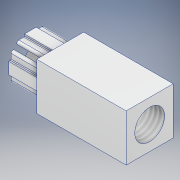
# Autodesk Inventor part: Line 5 Bucket Adapter
Saved by Autodesk Inventor 2020 (Build 240168000, 168)
## iProperties
Created: 2019-10-01
Part Number: Line 5 Bucket Adapter
Material: Aluminum 6061
Document SubType Name: Modeling
Designer: Matt
Density: 2.7 g/cm^3
Appearance: Aluminum - Flat
Mass: 38.6702 g
Surface Area: 66.6995 cm^2
Volume: 14.3223 cm^3
Author: Matt
Autodesk Inventor part; units mm, degrees
ref_plane "YZ Plane" through (0, 0, 0) normal (1, 0, 0) x (0, 1, 0)
ref_plane "XZ Plane" through (0, 0, 0) normal (0, 1, 0) x (-1, 0, 0)
ref_plane "XY Plane" through (0, 0, 0) normal (0, 0, 1) x (1, 0, 0)
sketch "Sketch1" plane through (0, 0, 0) normal (1, 0, 0) x (0, 1, 0)
  arc A0 (3.3, 10) -> (2.5, 9.2) centre (3.3, 9.2) ccw
  line L0 (2.5, 9.2) -> (2.5, 8.5)
  arc A1 (2.5, 8.5) -> (2.8, 8.2) centre (2.8, 8.5) ccw
  line L1 (2.8, 8.2) -> (4.9176, 8.2)
  arc A2 (5.5062, 6.779) -> (4.9176, 8.2) centre (4.9176, 7.3676) ccw
  line L2 (5.5062, 6.779) -> (3.2559, 4.5287)
  arc A3 (1.1346, 3.65) -> (3.2559, 4.5287) centre (1.1346, 6.65) ccw
  line L3 (1.1346, 3.65) -> (-1.1346, 3.65)
  arc A4 (-3.2559, 4.5287) -> (-1.1346, 3.65) centre (-1.1346, 6.65) ccw
  line L4 (-3.2559, 4.5287) -> (-5.5062, 6.779)
  arc A5 (-4.9176, 8.2) -> (-5.5062, 6.779) centre (-4.9176, 7.3676) ccw
  line L5 (-4.9176, 8.2) -> (-2.8, 8.2)
  arc A6 (-2.8, 8.2) -> (-2.5, 8.5) centre (-2.8, 8.5) ccw
  line L6 (-2.5, 8.5) -> (-2.5, 9.2)
  arc A7 (-2.5, 9.2) -> (-3.3, 10) centre (-3.3, 9.2) ccw
  line L7 (-8, 10) -> (-3.3, 10)
  arc A8 (-8, 10) -> (-10, 8) centre (-8, 8) ccw
  line L8 (-10, -3.3) -> (-10, 8)
  arc A9 (-10, 3.3) -> (-9.2, 2.5) centre (-9.2, 3.3) ccw
  line L9 (-9.2, 2.5) -> (-8.5, 2.5)
  arc A10 (-8.5, 2.5) -> (-8.2, 2.8) centre (-8.5, 2.8) ccw
  line L10 (-8.2, 2.8) -> (-8.2, 4.9176)
  arc A11 (-6.779, 5.5062) -> (-8.2, 4.9176) centre (-7.3676, 4.9176) ccw
  line L11 (-6.779, 5.5062) -> (-4.5287, 3.2559)
  arc A12 (-3.65, 1.1346) -> (-4.5287, 3.2559) centre (-6.65, 1.1346) ccw
  line L12 (-3.65, 1.1346) -> (-3.65, -1.1346)
  arc A13 (-4.5287, -3.2559) -> (-3.65, -1.1346) centre (-6.65, -1.1346) ccw
  line L13 (-4.5287, -3.2559) -> (-6.779, -5.5062)
  arc A14 (-8.2, -4.9176) -> (-6.779, -5.5062) centre (-7.3676, -4.9176) ccw
  line L14 (-8.2, -4.9176) -> (-8.2, -2.8)
  arc A15 (-8.2, -2.8) -> (-8.5, -2.5) centre (-8.5, -2.8) ccw
  line L15 (-8.5, -2.5) -> (-9.2, -2.5)
  arc A16 (-9.2, -2.5) -> (-10, -3.3) centre (-9.2, -3.3) ccw
  line L16 (-10, -8) -> (-10, -3.3)
  arc A17 (-10, -8) -> (-8, -10) centre (-8, -8) ccw
  line L17 (3.3, -10) -> (-8, -10)
  arc A18 (-3.3, -10) -> (-2.5, -9.2) centre (-3.3, -9.2) ccw
  line L18 (-2.5, -9.2) -> (-2.5, -8.5)
  arc A19 (-2.5, -8.5) -> (-2.8, -8.2) centre (-2.8, -8.5) ccw
  line L19 (-2.8, -8.2) -> (-4.9176, -8.2)
  arc A20 (-5.5062, -6.779) -> (-4.9176, -8.2) centre (-4.9176, -7.3676) ccw
  line L20 (-5.5062, -6.779) -> (-3.2559, -4.5287)
  arc A21 (-1.1346, -3.65) -> (-3.2559, -4.5287) centre (-1.1346, -6.65) ccw
  line L21 (-1.1346, -3.65) -> (1.1346, -3.65)
  arc A22 (3.2559, -4.5287) -> (1.1346, -3.65) centre (1.1346, -6.65) ccw
  line L22 (3.2559, -4.5287) -> (5.5062, -6.779)
  arc A23 (4.9176, -8.2) -> (5.5062, -6.779) centre (4.9176, -7.3676) ccw
  line L23 (4.9176, -8.2) -> (2.8, -8.2)
  arc A24 (2.8, -8.2) -> (2.5, -8.5) centre (2.8, -8.5) ccw
  line L24 (2.5, -8.5) -> (2.5, -9.2)
  arc A25 (2.5, -9.2) -> (3.3, -10) centre (3.3, -9.2) ccw
  line L25 (8, -10) -> (3.3, -10)
  arc A26 (8, -10) -> (10, -8) centre (8, -8) ccw
  line L26 (10, 3.3) -> (10, -8)
  arc A27 (10, -3.3) -> (9.2, -2.5) centre (9.2, -3.3) ccw
  line L27 (9.2, -2.5) -> (8.5, -2.5)
  arc A28 (8.5, -2.5) -> (8.2, -2.8) centre (8.5, -2.8) ccw
  line L28 (8.2, -2.8) -> (8.2, -4.9176)
  arc A29 (6.779, -5.5062) -> (8.2, -4.9176) centre (7.3676, -4.9176) ccw
  line L29 (6.779, -5.5062) -> (4.5287, -3.2559)
  arc A30 (3.65, -1.1346) -> (4.5287, -3.2559) centre (6.65, -1.1346) ccw
  line L30 (3.65, -1.1346) -> (3.65, 1.1346)
  arc A31 (4.5287, 3.2559) -> (3.65, 1.1346) centre (6.65, 1.1346) ccw
  line L31 (4.5287, 3.2559) -> (6.779, 5.5062)
  arc A32 (8.2, 4.9176) -> (6.779, 5.5062) centre (7.3676, 4.9176) ccw
  line L32 (8.2, 4.9176) -> (8.2, 2.8)
  arc A33 (8.2, 2.8) -> (8.5, 2.5) centre (8.5, 2.8) ccw
  line L33 (8.5, 2.5) -> (9.2, 2.5)
  arc A34 (9.2, 2.5) -> (10, 3.3) centre (9.2, 3.3) ccw
  line L34 (10, 8) -> (10, 3.3)
  arc A35 (10, 8) -> (8, 10) centre (8, 8) ccw
  line L35 (-3.3, 10) -> (8, 10)
  circle A36 centre (0, 0) radius 2.15
  line L36 (2.5, 9.2) -> (-2.5, 9.2)
  line L37 (-9.2, 2.5) -> (-9.2, -2.5)
  line L38 (-2.5, -9.2) -> (2.5, -9.2)
  line L39 (9.2, -2.5) -> (9.2, 2.5)
  point P0 (0, 0)
  point P1 (0, 0)
  point P2 (-9.2, 2.5)
  point P3 (-1.2, -12.5)
  point P4 (-2.5, -9.2)
  point P5 (10.5, -19.2)
  point P6 (17.2, -12.5)
  point P7 (9.2, 2.5)
  point P8 (9.2, -2.5)
  dimension "d2" = 360
  constraints: 80 end point, 72 point on circle, 37 centre point, 4 point on line, 1 coincident, 1 horizontal, 13 other
extrude "Extrusion1" add sketch "Sketch1" along normal blind 12.7 contours L0 A1 L1 A2 L2 A3 L3 A4 L4 A5 L5 A6 L6 L36 | L39 L27 A28 L28 A29 L29 A30 L30 A31 L31 A32 L32 A33 L33 | L9 A10 L10 A11 L11 A12 L12 A13 L13 A14 L14 A15 L15 L37 | L38 L18 A19 L19 A20 L20 A21 L21 A22 L22 A23 L23 A24 L24 | A36
sketch "Sketch2" plane through (12.7, 0, 0) normal (1, 0, 0) x (0, 0, -1)
  circle A0 centre (0, 0) radius 2.15 projected
  line L0 (-10, -10) -> (10, -10)
  line L1 (10, -10) -> (10, 10)
  line L2 (10, 10) -> (-10, 10)
  line L3 (-10, 10) -> (-10, -10)
  line L4 (-10, -10) -> (10, 10) construction
  line L5 (10, -10) -> (-10, 10) construction
  point P0 (0, 0)
  dimension "d6" = 20
  dimension "d7" = 20
  constraints: 12 end point, 2 midpoint, 2 parallel, 1 horizontal, 1 perpendicular
  measures "d6" distance of L2.end L1.end
  measures "d7" distance of L1.end L0.end
extrude "Extrusion2" add sketch "Sketch2" along normal blind 38.1
sketch "Sketch3" plane through (50.8, 0, 0) normal (1, 0, 0) x (0, 0, -1)
  circle A0 centre (0, 0) radius 6.35
  dimension "d10" = 12.7
  constraints: 1 centre point, 1 coincident
  measures "d10" diameter of A0
extrude "Extrusion3" cut sketch "Sketch3" against normal blind 25.4
thread "Thread1" size "1/2-13 UNC" class "2B" standard "ANSI Unified Screw Threads" full length
body "Solid1"
